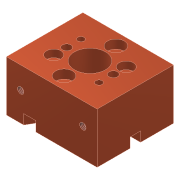
# Autodesk Inventor part: Part7
Saved by Autodesk Inventor 2022.4 (Build 264492000, 492)
## iProperties
Category: -
Company: Universiteit van Amsterdam
Created: 2023-08-21
Part Number: Part7
Material: Copper
Document SubType Name: Modeling
Designer: RbSrWorkstation1
Density: 8.94 g/cm^3
Appearance: Copper - Satin
User Status: Work in Progress
Author: RbSrWorkstation1
Revision Number: A
Autodesk Inventor part; units mm, degrees
ref_plane "YZ Plane" through (0, 0, 0) normal (1, 0, 0) x (0, 1, 0)
ref_plane "XZ Plane" through (0, 0, 0) normal (0, 1, 0) x (-1, 0, 0)
ref_plane "XY Plane" through (0, 0, 0) normal (0, 0, 1) x (1, 0, 0)
sketch "Sketch24" plane through (0, 0, 0) normal (0, 1, 0) x (-1, 0, 0)
  line L0 (-17.5, 14.75) -> (17.5, 14.75)
  line L1 (17.5, 14.75) -> (17.5, -14.75)
  line L2 (17.5, -14.75) -> (-17.5, -14.75)
  line L3 (-17.5, -14.75) -> (-17.5, 14.75)
  line L4 (-17.5, 14.75) -> (17.5, -14.75) construction
  line L5 (17.5, 14.75) -> (-17.5, -14.75) construction
  line L6 (-9.3, 8.2) -> (9.3, 8.2)
  line L7 (12.3, 5.2) -> (12.3, -5.2)
  line L8 (9.3, -8.2) -> (-9.3, -8.2)
  line L9 (-12.3, -5.2) -> (-12.3, 5.2)
  line L10 (-12.3, 8.2) -> (12.3, -8.2) construction
  line L11 (12.3, 8.2) -> (-12.3, -8.2) construction
  arc A0 (12.3, 5.2) -> (9.3, 8.2) centre (9.3, 5.2) ccw
  arc A1 (9.3, -8.2) -> (12.3, -5.2) centre (9.3, -5.2) ccw
  arc A2 (-12.3, -5.2) -> (-9.3, -8.2) centre (-9.3, -5.2) ccw
  arc A3 (-9.3, 8.2) -> (-12.3, 5.2) centre (-9.3, 5.2) ccw
  circle A4 centre (0, 0) radius 12.25
  dimension "d54" = 35
  dimension "d55" = 29.5
  dimension "d56" = 16.4
  dimension "d57" = 24.6
  dimension "d58" = 3
  dimension "d59" = 24.5
  constraints: 24 end point, 8 point on circle, 8 point on line, 8 tangent, 5 centre point, 4 midpoint, 4 parallel, 3 equal radius, 2 horizontal, 2 perpendicular, 1 coincident
  measures "d54" distance of L1.end L2.end
  measures "d55" distance of L0.end L1.end
  measures "d56" distance between parallel lines of L8 L6
  measures "d57" distance of L10.end L11.end
  measures "d58" radius of A0
  measures "d59" diameter of A4
extrude "Extrusion20" add sketch "Sketch24" along normal blind 19.5 contours L0 L1 L2 L3 | L6 A4 L8 A2 L9 A3 | A4 L6 | L6 A4 L8 | L6 A0 L7 A1 L8 A4 | L8 A4
extrude "Extrusion21" cut sketch "Sketch24" along normal blind 3.8 contours L6 A4 L8 A2 L9 A3 | L6 A4 L8 | L6 A0 L7 A1 L8 A4
sketch "Sketch25" plane through (0, 19.5, 0) normal (0, 1, 0) x (1, 0, 0)
  line L0 (9, 5) -> (-9, -5) construction
  point P0 (0, 0)
  point P1 (9, -5)
  point P2 (-9, 5)
  point P3 (0, 0)
  dimension "d71" = 10
  dimension "d72" = 18
  constraints: 2 end point, 2 horizontal alignment, 2 vertical alignment, 1 coincident, 1 midpoint
  measures "d71" distance of point (9, -5) L0.start
  measures "d72" distance of point (-9, 5) L0.start
hole "Hole1" at (9, 19.5, -5) at (-9, 19.5, 5) direction (0, -1, 0) diameter 2.6 end through all counterbore diameter 5.5 counterbore depth 2.9 clearance for "Socket Head Cap Screw ISO 4762" size "M2.5" standard "ISO"
sketch "Sketch26" plane through (0, 3.8, 0) normal (0, -1, 0) x (1, 0, 0)
  circle A0 centre (0, 0) radius 6
  dimension "d73" = 12
  constraints: 1 centre point, 1 coincident
  measures "d73" diameter of A0
extrude "Extrusion22" cut sketch "Sketch26" against normal through all
sketch "Sketch27" plane through (-17.5, 0, 14.75) normal (0, 0, 1) x (1, 0, 0)
  line L0 (0, 0) -> (35, 0) projected
  line L1 (0, 19.5) -> (35, 19.5) projected
  point P0 (17.5, 0)
  point P1 (29.5, 11)
  point P2 (5.5, 11)
  point P3 (17.5, 0)
  point P4 (17.5, 0)
  point P5 (0, 11)
  dimension "d83" = 12
  dimension "d84" = 12
  dimension "d145" = 8.5
  constraints: 2 horizontal alignment, 2 midpoint
  measures "d83" horizontal distance of point (17.5, 0) point (29.5, 11)
  measures "d84" horizontal distance of point (17.5, 0) point (5.5, 11)
  measures "d145" distance from line of point (5.5, 11) L1
hole "Hole2" at (12, 11, 14.75) at (-12, 11, 14.75) direction (0, 0, -1) diameter 2.459 depth 9 tip angle 118 thread size "M3x0.5" class "6H" standard "ISO Metric profile"
sketch "Sketch28" plane through (17.5, 0, -14.75) normal (0, 0, -1) x (-1, 0, 0)
  circle A0 centre (29.5, 11) radius 1.2295 projected
  circle A1 centre (5.5, 11) radius 1.2295 projected
  point P0 (17.5, 0)
  constraints: 2 coincident
hole "Hole3" at (-12, 11, -14.75) at (12, 11, -14.75) direction (0, 0, 1) diameter 2.459 depth 9 tip angle 118 thread size "M3x0.5" class "6H" standard "ISO Metric profile"
sketch "Sketch29" plane through (0, 3.8, 0) normal (0, -1, 0) x (1, 0, 0)
  line L0 (-9, -5.5) -> (-9, 1.5) construction
  line L1 (-7.5, -5.5) -> (-7.5, 1.5)
  line L2 (-10.5, 1.5) -> (-10.5, -5.5)
  arc A0 (-10.5, -5.5) -> (-7.5, -5.5) centre (-9, -5.5) ccw
  arc A1 (-7.5, 1.5) -> (-10.5, 1.5) centre (-9, 1.5) ccw
  line L3 (9, -1.5) -> (9, 5.5) construction
  line L4 (10.5, -1.5) -> (10.5, 5.5)
  line L5 (7.5, 5.5) -> (7.5, -1.5)
  arc A2 (7.5, -1.5) -> (10.5, -1.5) centre (9, -1.5) ccw
  arc A3 (10.5, 5.5) -> (7.5, 5.5) centre (9, 5.5) ccw
  point P0 (0, 0)
  point P1 (-9, -2)
  point P2 (9, 2)
  point P3 (-9, 3)
  point P4 (-9, -7)
  dimension "d94" = 3
  dimension "d95" = 10
  dimension "d96" = 1.5
  dimension "d97" = 9
  dimension "d98" = 9
  dimension "d99" = 1.5
  constraints: 16 end point, 10 point on circle, 8 tangent, 4 centre point, 4 parallel, 2 midpoint, 1 equal radius, 1 vertical
  measures "d94" distance between parallel lines of L1 L2
  measures "d95" distance of point (-9, 3) point (-9, -7)
  measures "d96" vertical distance of point (0, 0) L2.start
  measures "d97" distance from line of point (0, 0) L0
  measures "d98" distance from line of point (0, 0) L3
  measures "d99" vertical distance of L3.start point (0, 0)
extrude "Extrusion23" cut sketch "Sketch29" against normal blind 2.5
sketch "Sketch30" plane through (0, 6.3, 0) normal (0, -1, 0) x (1, 0, 0)
  arc A0 (-10.5, -5.5) -> (-7.5, -5.5) centre (-9, -5.5) ccw projected
  arc A1 (10.5, 5.5) -> (7.5, 5.5) centre (9, 5.5) ccw projected
  point P0 (0, 0)
  constraints: 2 coincident
hole "Hole4" at (-9, 6.3, -5.5) at (9, 6.3, 5.5) direction (0, 1, 0) diameter 2.5 end through all
sketch "Sketch31" plane through (0, 6.3, 0) normal (0, -1, 0) x (1, 0, 0)
  arc A0 (-7.5, 1.5) -> (-10.5, 1.5) centre (-9, 1.5) ccw projected
  arc A1 (7.5, -1.5) -> (10.5, -1.5) centre (9, -1.5) ccw projected
  point P0 (0, 0)
  point P1 (-9, 0)
  point P2 (9, 0)
  point P3 (9, 0)
  point P4 (-9, 3)
  constraints: 2 horizontal alignment, 2 vertical alignment, 1 coincident, 1 point on circle
hole "Hole5" at (-9, 6.3, 0) at (9, 6.3, 0) direction (0, 1, 0) diameter 2.013 end through all thread size "M2.5x0.45" class "6H" standard "ISO Metric profile"
sketch "Sketch32" plane through (0, 19.5, 0) normal (0, 1, 0) x (1, 0, 0)
  circle A0 centre (-9, 0) radius 1.0065 projected
  circle A1 centre (9, 0) radius 1.0065 projected
  point P0 (0, 0)
  point P1 (-9.5915, -2.3144)
  point P2 (-8.4085, -2.3144)
  point P3 (9.5915, 2.3144)
  point P4 (8.4085, 2.3144)
  constraints: 2 coincident, 2 other
hole "Hole6" at (-9, 19.5, 0) at (9, 19.5, 0) direction (0, -1, 0) diameter 3.3 depth 7 tip angle 118
sketch "Sketch33" plane through (0, 19.5, 0) normal (0, 1, 0) x (1, 0, 0)
  point P0 (0, 0)
  point P1 (0, -10)
  point P2 (0, 10)
  dimension "d131" = 10
  dimension "d132" = 10
  constraints: 2 vertical alignment
  measures "d131" distance of point (0, -10) point (0, 0)
  measures "d132" distance of point (0, 0) point (0, 10)
hole "Hole7" at (0, 19.5, 10) at (0, 19.5, -10) direction (0, -1, 0) diameter 3.1 end through all counterbore diameter 6.5 counterbore depth 3.4 clearance for "Socket Head Cap Screw ISO 4762" size "M3" standard "ISO"
sketch "Sketch35" plane through (0, 0, 0) normal (0, -1, 0) x (1, 0, 0)
  line L0 (50, -2) -> (0, -2)
  line L1 (0, -2) -> (0, 2)
  line L2 (0, 2) -> (50, 2)
  line L3 (50, 2) -> (50, -2)
  point P0 (0, 0)
  point P1 (0, 0)
  dimension "d138" = 4
  dimension "d139" = 50
  constraints: 8 end point, 2 parallel, 1 coincident, 1 horizontal, 1 midpoint, 1 perpendicular
  measures "d138" distance of L2.end L0.start
  measures "d139" distance of L0.start L0.end
extrude "Extrusion24" cut sketch "Sketch35" against normal blind 3.8
pattern_circular "Circular Pattern1" count 3 over 360 about axis through (0, 3.8, 0) along (0, 1, 0) of "Extrusion24"
body "Solid2"
